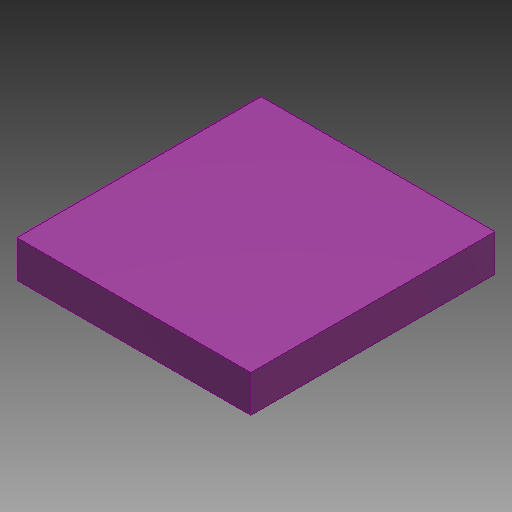
# Autodesk Inventor part: REG1117
Saved by Autodesk Inventor 2017.3 (Build 213256000, 256)
## iProperties
Part Number: REG1117
Material: Generisch
Document SubType Name: Modeling
Designer: Nils
Density: 1 g/cm^3
Appearance: SOT223, REG1117
Author: Nils
Autodesk Inventor part; units mm, degrees
ref_plane "YZ Plane" through (0, 0, 0) normal (1, 0, 0) x (0, 1, 0)
ref_plane "XZ Plane" through (0, 0, 0) normal (0, 1, 0) x (-1, 0, 0)
ref_plane "XY Plane" through (0, 0, 0) normal (0, 0, 1) x (1, 0, 0)
sketch "SOT223, REG1117_21" plane through (0, 0, 0) normal (0, 0, 1) x (1, 0, 0)
  line L0 (-3.2002, 3.302) -> (3.124, 3.302)
  line L1 (3.124, 3.302) -> (3.124, -3.302)
  line L2 (3.124, -3.302) -> (-3.2002, -3.302)
  line L3 (-3.2002, -3.302) -> (-3.2002, 3.302)
  constraints: 8 end point
extrude "Extrusion1" add sketch "SOT223, REG1117_21" along normal blind 1
